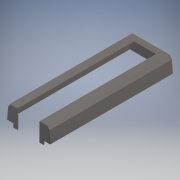
# Autodesk Inventor part: PRZEDNIA CZARNA OBUDOWA STOJAKA
Saved by Autodesk Inventor 2017 SP1 (Build 210196100, 196)
## iProperties
Created: 2020-12-27
Part Number: PRZEDNIA CZARNA OBUDOWA STOJAKA
Material: Tworzywo sztuczne, nieprzezroczyste czarne
Document SubType Name: Modeling
Designer: Napoleon
Mass: 18.6576 g
Surface Area: 302.502 cm^2
Volume: 19.5983 cm^3
Density: 0.952 g/cm^3
Appearance: Chropowaty, teksturowany - czarny
Author: Napoleon
Autodesk Inventor part; units mm, degrees
ref_plane "YZ Plane" through (0, 0, 0) normal (1, 0, 0) x (0, 1, 0)
ref_plane "XZ Plane" through (0, 0, 0) normal (0, 1, 0) x (-1, 0, 0)
ref_plane "XY Plane" through (0, 0, 0) normal (0, 0, 1) x (1, 0, 0)
sketch "Szkic1" plane through (0, 0, 0) normal (0, 0, 1) x (1, 0, 0)
  line L0 (72.8864, 226.5) -> (7.8864, 226.5)
  line L1 (7.8864, 226.5) -> (7.8864, 42.5)
  line L2 (72.8864, 42.5) -> (72.8864, 226.5)
  line L3 (9.3864, 225) -> (71.3864, 225)
  line L4 (9.3864, 44) -> (9.3864, 225)
  line L5 (71.3864, 225) -> (71.3864, 44)
  line L6 (7.8864, 42.5) -> (23.8864, 42.5)
  line L7 (9.3864, 44) -> (23.8864, 44)
  line L8 (23.8864, 44) -> (23.8864, 42.5)
  line L9 (72.8864, 42.5) -> (56.8864, 42.5)
  line L10 (71.3864, 44) -> (56.8864, 44)
  line L11 (56.8864, 44) -> (56.8864, 42.5)
  point P0 (0, 0)
  constraints: 24 end point, 2 horizontal, 1 perpendicular
extrude "Wyciągnięcie proste1" add sketch "Szkic1" along normal blind 22
sketch "Szkic2" plane through (7.8864, 226.5, 0) normal (0, 1, 0) x (1, 0, 0)
  line L0 (0, 0) -> (1, -17)
  line L1 (60.5, -22) -> (4.5, -22)
  line L2 (60.05, -20.5) -> (4.9345, -20.5)
  line L3 (0, 0) -> (1.5, 0)
  line L4 (1.5, 0) -> (2.5, -17)
  line L5 (4.5, -22) -> (1, -17)
  line L6 (65, 0) -> (64, -17)
  line L7 (63.5, 0) -> (62.5, -17)
  line L8 (60.5, -22) -> (64, -17)
  line L9 (62.5, -17) -> (60.05, -20.5)
  line L10 (2.5, -17) -> (4.9345, -20.5)
  line L11 (63.5, 0) -> (65, 0)
  point P0 (-7.8864, 0)
  dimension "d13" = 1.5
  constraints: 24 end point, 1 horizontal, 1 parallel
  measures "d13" distance of L0.start L3.end
extrude "Wyciągnięcie proste2" add sketch "Szkic2" against normal up to surface (184 mm away)
sketch "Szkic3" plane through (7.8864, 226.5, 0) normal (0, 1, 0) x (1, 0, 0)
  line L0 (65, 0) -> (65, -22)
  line L1 (63.5, -17.5) -> (65, 0)
  line L2 (60.5, -22) -> (63.5, -17.5)
  line L3 (65, -22) -> (60.5, -22)
  line L4 (0, 0) -> (0, -22)
  line L5 (1.5, -17.5) -> (0, 0)
  line L6 (4.5, -22) -> (1.5, -17.5)
  line L7 (0, -22) -> (4.5, -22)
  line L8 (0, 0) -> (0, -22)
  line L9 (65, -22) -> (0, -22)
  line L10 (65, 0) -> (0, 0)
  constraints: 22 end point
extrude "Wyciągnięcie proste3" cut sketch "Szkic3" against normal up to surface (184 mm away) contours L0 L3 L2 L1 | L5 L6 L7 L4
sketch "Szkic4" plane through (0, 0, 22) normal (0, 0, 1) x (1, 0, 0)
  line L0 (68.3864, 226.5) -> (12.3864, 226.5) projected
  line L1 (12.3864, 42.5) -> (68.3864, 42.5) projected
  line L2 (23.8864, 44) -> (23.8864, 42.5) projected
  line L3 (23.8864, 42.5) -> (23.8864, 216.5)
  line L4 (23.8864, 42.5) -> (197.8864, 42.5) construction
  line L5 (23.8864, 216.5) -> (56.8864, 216.5)
  line L6 (56.8864, 42.5) -> (23.8864, 42.5) projected
  line L7 (56.8864, 216.5) -> (56.8864, 42.5)
  line L8 (56.8864, 42.5) -> (23.8864, 42.5)
  point P0 (66.8864, 42.5)
  point P1 (66.8864, 226.5)
  point P2 (13.8864, 226.5)
  point P3 (13.8864, 42.5)
  point P4 (0, 0)
  dimension "d18" = 174
  dimension "d19" = 90
  dimension "d20" = 33
  dimension "d21" = 90
  constraints: 10 end point, 3 perpendicular, 1 collinear, 1 horizontal
  measures "d18" distance of L2.end L3.end
  measures "d19" angle of L4 L3
  measures "d20" distance of L3.end L5.end
  measures "d21" angle of L5 L7
extrude "Wyciągnięcie proste4" cut sketch "Szkic4" against normal through all
sketch "Szkic5" plane through (0, 0, 0) normal (0, 0, -1) x (-1, 0, 0)
  line L0 (-17.8864, 42.5) -> (-17.8864, 44) projected
  line L1 (-62.8864, 44) -> (-62.8864, 42.5) projected
  line L2 (-62.8864, 44) -> (-56.8864, 44)
  line L3 (-56.8864, 44) -> (-56.8864, 42.5)
  line L4 (-56.8864, 42.5) -> (-62.8864, 42.5)
  line L5 (-62.8864, 42.5) -> (-62.8864, 44)
  line L6 (-23.8864, 44) -> (-17.8864, 44)
  line L7 (-17.8864, 44) -> (-17.8864, 42.5)
  line L8 (-17.8864, 42.5) -> (-23.8864, 42.5)
  line L9 (-23.8864, 42.5) -> (-23.8864, 44)
  point P0 (0, 0)
  constraints: 16 end point, 4 parallel, 2 horizontal, 2 perpendicular
extrude "Wyciągnięcie proste5" add sketch "Szkic5" along normal up to surface (6.0684 mm away)
sketch "Szkic6" plane through (23.8864, 44, -6.0684) normal (0, 0, -1) x (-1, 0, 0)
  line L0 (6, 0) -> (6, -1.5) projected
  line L1 (0, 0) -> (6, 0) projected
  line L2 (0, -1.5) -> (0, 0) projected
  line L3 (6, -1.5) -> (0, -1.5) projected
  line L4 (-39, 0) -> (-39, -1.5) projected
  line L5 (-33, 0) -> (-33, -1.5) projected
  line L6 (-39, 0) -> (-33, 0) projected
  line L7 (-33, -1.5) -> (-39, -1.5) projected
  point P0 (23.8864, -44)
extrude "Wyciągnięcie proste6" cut sketch "Szkic6" against normal blind 0.5
fillet "Zaokrąglenie2" radius 1 11 edges at (72.1364, 42.5, 8.75) (69.8864, 42.5, 19.75) (62.6364, 42.5, 22) (18.1364, 42.5, 22) (10.8864, 42.5, 19.75) (8.6364, 42.5, 8.75) (72.1364, 226.5, 8.75) (69.8864, 226.5, 19.75) (40.3864, 226.5, 22) (10.8864, 226.5, 19.75) (8.6364, 226.5, 8.75)
